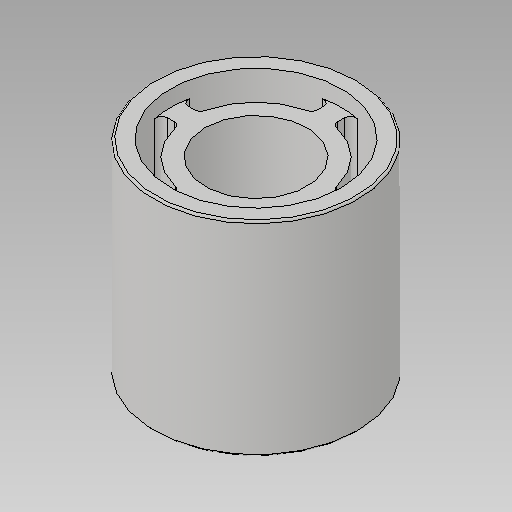
# Autodesk Inventor part: beam_single_1x1_part
Saved by Autodesk Inventor 2020 (Build 240168000, 168)
## iProperties
Created: 2019-04-27
Part Number: beam_single_1x1_part
Material: Generic
Document SubType Name: Modeling
Designer: Varga Daniel
Density: 1 g/cm^3
Appearance: Default
Author: Varga Daniel
Autodesk Inventor part; units mm, degrees
ref_plane "YZ Plane" through (0, 0, 0) normal (1, 0, 0) x (0, 1, 0)
ref_plane "XZ Plane" through (0, 0, 0) normal (0, 1, 0) x (-1, 0, 0)
ref_plane "XY Plane" through (0, 0, 0) normal (0, 0, 1) x (1, 0, 0)
derived "Base_part.ipt"
sketch "Beam_sketch" plane through (0, 0, 0) normal (0, 1, 0) x (-1, 0, 0)
  circle A0 centre (0, 0) radius 2.5
  line L0 (0, 0) -> (0, -5.5751) construction
  line L1 (3.6649, 0) -> (-4.8297, 0) construction
  arc A1 (-5, 0) -> (0, -5) centre (0, 0) ccw
  line L2 (0, -5) -> (5, -5)
  line L3 (-5, 0) -> (-5, 5)
  line L4 (-5, 5) -> (5, 5)
  line L5 (5, 5) -> (5, -5)
  line L6 (0.5, -3.4641) -> (0.5, -4)
  line L7 (-0.5, -3.2619) -> (-0.5, -4)
  line L8 (0.5, 3.4641) -> (0.5, 4)
  line L9 (-0.5, 3.4641) -> (-0.5, 4)
  line L10 (3.4641, -0.5) -> (4, -0.5)
  line L11 (3.4641, 0.5) -> (4, 0.5)
  line L12 (-3.2619, -0.5) -> (-4, -0.5)
  line L13 (-3.4641, 0.5) -> (-4, 0.5)
  line L14 (-0.5, -4) -> (4, -4)
  arc A2 (-0.5, 3.4641) -> (-3.4641, 0.5) centre (0, 0) ccw
  arc A3 (-3.2619, -0.5) -> (-0.5, -3.2619) centre (0, 0) ccw
  arc A4 (-4.1701, -0.5) -> (-0.5, -4.1701) centre (0, 0) ccw
  line L15 (4, -4) -> (4, -0.5)
  line L16 (4, -0.5) -> (4, 4)
  line L17 (4, 4) -> (0.5, 4)
  line L18 (0.5, 4) -> (-4, 4)
  line L19 (-4, 4) -> (-4, -0.5)
  arc A5 (0.5, -3.4641) -> (3.4641, -0.5) centre (0, 0) ccw
  arc A6 (3.4641, 0.5) -> (0.5, 3.4641) centre (0, 0) ccw
  line L20 (-4, -0.5) -> (-4.1701, -0.5)
  line L21 (-0.5, -4) -> (-0.5, -4.1701)
sketch "Sketch3" plane through (0, 0, 0) normal (0, 1, 0) x (-1, 0, 0)
  circle A0 centre (0, 0) radius 2.5 projected
  line L0 (0, 0) -> (0, -5.5751) construction
  line L1 (3.6649, 0) -> (-4.8297, 0) construction
  arc A1 (-3.2619, -0.5) -> (-0.5, -3.2619) centre (0, 0) ccw projected
  line L2 (-0.5, -3.2619) -> (-0.5, -4) projected
  line L3 (-0.5, -4) -> (-0.5, -4.1701) projected
  arc A2 (-4.1701, -0.5) -> (-0.5, -4.1701) centre (0, 0) ccw projected
  line L4 (-3.2619, -0.5) -> (-4, -0.5) projected
  line L5 (-4, -0.5) -> (-4.1701, -0.5) projected
  arc A3 (-5, 0) -> (0, -5) centre (0, 0) ccw projected
  arc A4 (0.5, -3.2619) -> (3.2619, -0.5) centre (0, 0) ccw
  line L6 (0.5, -3.2619) -> (0.5, -4)
  line L7 (0.5, -4) -> (0.5, -4.1701)
  arc A5 (0.5, -4.1701) -> (4.1701, -0.5) centre (0, 0) ccw
  line L8 (3.2619, -0.5) -> (4, -0.5)
  line L9 (4, -0.5) -> (4.1701, -0.5)
  arc A6 (0, -5) -> (5, 0) centre (0, 0) ccw
  line L10 (0, 0) -> (0, 5.5751) construction
  arc A7 (-0.5, 3.2619) -> (-3.2619, 0.5) centre (0, 0) ccw
  line L11 (-0.5, 3.2619) -> (-0.5, 4)
  line L12 (-0.5, 4) -> (-0.5, 4.1701)
  arc A8 (-0.5, 4.1701) -> (-4.1701, 0.5) centre (0, 0) ccw
  line L13 (-3.2619, 0.5) -> (-4, 0.5)
  line L14 (-4, 0.5) -> (-4.1701, 0.5)
  arc A9 (0, 5) -> (-5, 0) centre (0, 0) ccw
  arc A10 (3.2619, 0.5) -> (0.5, 3.2619) centre (0, 0) ccw
  line L15 (0.5, 3.2619) -> (0.5, 4)
  line L16 (0.5, 4) -> (0.5, 4.1701)
  circle A11 centre (0, 0) radius 4.2
  line L17 (3.2619, 0.5) -> (4, 0.5)
  line L18 (4, 0.5) -> (4.1701, 0.5)
  arc A12 (5, 0) -> (0, 5) centre (0, 0) ccw
  point P0 (4.8297, 0)
  constraints: 26 end point, 22 point on circle, 22 symmetric about line, 9 centre point, 9 other
extrude "Extrusion1" add sketch "Sketch3" along normal mid plane 10 contours A9 A12 A6 A3
extrude "Extrusion2" add sketch "Sketch3" along normal mid plane 8.4 contours L4 L5 A11 L14 L13 A7 L11 L12 L16 L15 A10 L17 L18 L9 L8 A4 L6 L7 L3 L2 A1
extrude "Extrusion3" add sketch "Sketch3" along normal mid plane 1 contours A1 L2 L3 A2 L5 L4 | A8 L12 L11 A7 L13 L14 | L7 L6 A4 L8 L9 A5 | A11 L18 L17 A10 L15 L16
fillet "Fillet1" radius 0.3 32 edges at (0.5, 2.35, 3.2619) (0.5, 2.35, 4.1701) (3.2619, 2.35, 0.5) (4.1701, 2.35, 0.5) (3.2619, 2.35, -0.5) (4.1701, 2.35, -0.5) (0.5, 2.35, -3.2619) (0.5, 2.35, -4.1701) (-0.5, 2.35, -3.2619) (-0.5, 2.35, -4.1701) (-3.2619, 2.35, -0.5) (-4.1701, 2.35, -0.5) (-4.1701, 2.35, 0.5) (-3.2619, 2.35, 0.5) (-0.5, 2.35, 4.1701) (-0.5, 2.35, 3.2619) (0.5, -2.35, 3.2619) (0.5, -2.35, 4.1701) (-0.5, -2.35, 4.1701) (-0.5, -2.35, 3.2619) (-3.2619, -2.35, 0.5) (-4.1701, -2.35, 0.5) (-3.2619, -2.35, -0.5) (-4.1701, -2.35, -0.5) (-0.5, -2.35, -3.2619) (-0.5, -2.35, -4.1701) (0.5, -2.35, -4.1701) (0.5, -2.35, -3.2619) (3.2619, -2.35, -0.5) (4.1701, -2.35, -0.5) (4.1701, -2.35, 0.5) (3.2619, -2.35, 0.5)
fillet "Fillet2" radius 0.1 8 edges at (3.5355, -5, 3.5355) (-3.5355, -5, 3.5355) (3.5355, -5, -3.5355) (-3.5355, -5, -3.5355) (3.5355, 5, 3.5355) (-3.5355, 5, 3.5355) (3.5355, 5, -3.5355) (-3.5355, 5, -3.5355)
equation "\"d1\" = Overall_height"
equation "\"d3\" = Hole_height"
equation "\"d5\" = Inner_height"
equation "\"d7\" = Inner_fillet"
equation "\"d8\" = Outer_edge_fillet"
equation "\"Overall_height\" = 10"
equation "\"Hole_height\" = 8.4"
equation "\"Inner_height\" = 1"
equation "\"Inner_fillet\" = 0.3"
equation "\"Outer_edge_fillet\" = 0.1"
body "Solid1"
